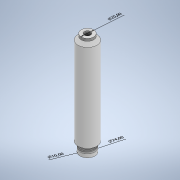
# Autodesk Inventor part: Manche interm
Saved by Autodesk Inventor 2021 (Build 250183000, 183)
## iProperties
Created: 2020-09-18
Part Number: Manche interm
Material: Générique
Document SubType Name: Modeling
Designer: Utilisateur
Density: 1 g/cm^3
Appearance: Par défaut
Author: Utilisateur
Autodesk Inventor part; units mm, degrees
ref_plane "YZ Plane" through (0, 0, 0) normal (1, 0, 0) x (0, 1, 0)
ref_plane "XZ Plane" through (0, 0, 0) normal (0, 1, 0) x (-1, 0, 0)
ref_plane "XY Plane" through (0, 0, 0) normal (0, 0, 1) x (1, 0, 0)
sketch "Esquisse1" plane through (0, 0, 0) normal (0, 1, 0) x (-1, 0, 0)
  circle A0 centre (0, 0) radius 15
  dimension "d0" = 30
  constraints: 1 centre point, 1 coincident
  measures "d0" diameter of A0
extrude "Extrusion1" add sketch "Esquisse1" along normal blind 150
sketch "Esquisse2" plane through (0, 0, 0) normal (0, 1, 0) x (-1, 0, 0)
  circle A0 centre (0, 0) radius 10
  dimension "d5" = 20
  constraints: 1 centre point, 1 coincident
  measures "d5" diameter of A0
extrude "Extrusion2" add sketch "Esquisse2" along normal blind 154 and the other way blind 5
thread "Filetage2" size "M17x1.5" class "6g" standard "ANSI Metric M Profile" length 4
chamfer "Chanfrein1" distance 5 angle 45 1 edges at (15, 150, 0)
chamfer "Chanfrein2" distance 5 angle 45 1 edges at (15, 0, 0)
sketch "Esquisse5" plane through (0, -5, 0) normal (0, -1, 0) x (1, 0, 0)
  circle A0 centre (0, 0) radius 12
  dimension "d24" = 24
  constraints: 1 centre point, 1 coincident
  measures "d24" diameter of A0
extrude "Extrusion4" add sketch "Esquisse5" along normal blind 5 and the other way blind 5
sketch "Esquisse3" plane through (0, 0, 0) normal (0, 1, 0) x (-1, 0, 0)
  circle A0 centre (0, 0) radius 10 projected
  circle A1 centre (0, 0) radius 5
  dimension "d33" = 10
  constraints: 1 centre point, 1 coincident
  measures "d33" diameter of A1
extrude "Extrusion3" cut sketch "Esquisse3" along normal blind 154 and the other way blind 72 contours A1
thread "Filetage5" size "M24x3" class "6g" standard "ANSI Metric M Profile" length 5 offset 5
